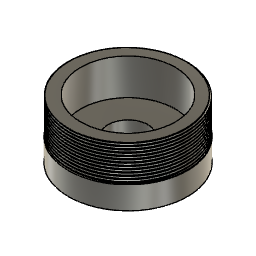
slide fit Powell mount (Autodesk Fusion 360 design; units mm, degrees)
Autodesk Fusion 360 part; units mm, degrees
cylinder "CylinderPrimitive7" add diameter 25.4 height 8 placed x (1, 0, 0) y (0, 1, 0) z (0, 0, 1) at (0, 0, 0) makes body 1
cylinder "CylinderPrimitive8" add diameter 26.4 height 5 placed x (1, 0, 0) y (0, 1, 0) z (0, 0, 1) at (0, 0, 8) separate body makes body 2
thread "Thread3" "ARC Optic Threads 1.035 Thor SM1 1.035-40 2A" major diameter 26.195 minor diameter 25.5727 pitch 0.635 angle 60 modelled right hand crest width 0.099 on face at (12.6369, -1.2645, 5.3333) crest through (13.0975, 0, -0.1588) on bodies 1
combine "Combine3" operation add target body 2 tool bodies 1
move_body "Move1" bodies 2 to x (1, 0, 0) y (0, -1, 0) z (0, 0, -1) at (0, 0, 13)
cylinder "CylinderPrimitive10" add diameter 21 height 8 placed x (1, 0, 0) y (0, 1, 0) z (0, 0, 1) at (0, 0, 13) separate body makes body 3
move_body "Move3" bodies 3 to x (1, 0, 0) y (0, 1, 0) z (0, 0, 1) at (0, 0, -8)
combine "Combine4" operation cut target body 2 tool bodies 3
cylinder "CylinderPrimitive11" cut diameter 8.9 height 5 placed x (1, 0, 0) y (0, 1, 0) z (0, 0, 1) at (0, 0, 0) bodies 2
